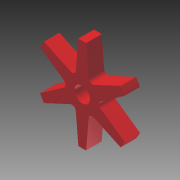
# Autodesk Inventor part: rubber intake star
Saved by Autodesk Inventor 2012 (Build 160160000, 160)
## iProperties
Created: 2013-07-07
Part Number: rubber intake star
Material: Default
Document SubType Name: Modeling
Designer: Bryce
Density: 1 g/cm^3
Author: Bryce
Autodesk Inventor part; units mm, degrees
ref_plane "YZ Plane" through (0, 0, 0) normal (1, 0, 0) x (0, 1, 0)
ref_plane "XZ Plane" through (0, 0, 0) normal (0, 1, 0) x (-1, 0, 0)
ref_plane "XY Plane" through (0, 0, 0) normal (0, 0, 1) x (1, 0, 0)
sketch "Sketch1" plane through (0, 0, 0) normal (0, 0, 1) x (1, 0, 0)
  arc A0 (3.175, 37.9675) -> (-3.175, 37.9675) centre (0, 0) ccw
  line L0 (-3.175, 37.9675) -> (-5.6418, 9.7719)
  line L1 (0, 38.1) -> (0, 0) construction
  arc A1 (-3.175, 37.9675) -> (-31.2933, 21.7334) centre (0, 0) ccw construction
  line L2 (-5.6418, 9.7719) -> (5.6418, 9.7719) construction
  line L3 (5.6418, 9.7719) -> (11.2836, 0) construction
  line L4 (11.2836, 0) -> (5.6418, -9.7719) construction
  line L5 (5.6418, -9.7719) -> (-5.6418, -9.7719) construction
  line L6 (-5.6418, -9.7719) -> (-11.2836, 0) construction
  line L7 (-11.2836, 0) -> (-5.6418, 9.7719) construction
  line L8 (3.175, 37.9675) -> (5.6418, 9.7719)
  line L9 (0, 0) -> (-32.9956, 19.05) construction
  line L10 (0, 0) -> (32.9956, 19.05) construction
  line L11 (0, 0) -> (-32.9956, -19.05) construction
  line L12 (0, 0) -> (32.9956, -19.05) construction
  line L13 (0, 0) -> (0, -38.1) construction
  line L14 (5.6418, 9.7719) -> (31.2933, 21.7334)
  line L15 (11.2836, 0) -> (34.4683, 16.2341)
  line L16 (11.2836, 0) -> (34.4683, -16.2341)
  line L17 (5.6418, -9.7719) -> (31.2933, -21.7334)
  arc A2 (31.2933, 21.7334) -> (3.175, 37.9675) centre (0, 0) ccw construction
  arc A3 (34.4683, 16.2341) -> (31.2933, 21.7334) centre (0, 0) ccw
  arc A4 (34.4683, -16.2341) -> (34.4683, 16.2341) centre (0, 0) ccw construction
  arc A5 (31.2933, -21.7334) -> (34.4683, -16.2341) centre (0, 0) ccw
  line L18 (5.6418, -9.7719) -> (3.175, -37.9675)
  line L19 (-5.6418, -9.7719) -> (-3.175, -37.9675)
  line L20 (-5.6418, -9.7719) -> (-31.2933, -21.7334)
  line L21 (-11.2836, 0) -> (-34.4683, -16.2341)
  line L22 (-11.2836, 0) -> (-34.4683, 16.2341)
  line L23 (-5.6418, 9.7719) -> (-31.2933, 21.7334)
  arc A6 (-31.2933, 21.7334) -> (-34.4683, 16.2341) centre (0, 0) ccw
  arc A7 (-34.4683, 16.2341) -> (-34.4683, -16.2341) centre (0, 0) ccw construction
  arc A8 (-34.4683, -16.2341) -> (-31.2933, -21.7334) centre (0, 0) ccw
  arc A9 (-31.2933, -21.7334) -> (-3.175, -37.9675) centre (0, 0) ccw construction
  arc A10 (-3.175, -37.9675) -> (3.175, -37.9675) centre (0, 0) ccw
  arc A11 (3.175, -37.9675) -> (31.2933, -21.7334) centre (0, 0) ccw construction
  circle A12 centre (0, 0) radius 6.35
  dimension "d10" = 38.1
  dimension "d1" = 6.35
  dimension "d2" = 3.175
  dimension "d3" = 5
  dimension "d5" = 5
  dimension "d6" = 5
  dimension "d7" = 5
  dimension "d8" = 5
  dimension "d9" = 5
  dimension "d13" = 12.7
  constraints: 48 end point, 47 point on circle, 10 centre point, 7 equal length, 3 coincident, 2 perpendicular, 1 collinear, 1 horizontal, 1 vertical, 49 other
  measures "d1" distance of L8.start L0.start
  measures "d2" horizontal distance of L1.start L0.start
  measures "d3" angle of L1 L0
  measures "d5" angle of L10 L14
  measures "d6" angle of L10 L15
  measures "d7" angle of L12 L16
  measures "d8" angle of L12 L17
  measures "d9" angle of L13 L19
  measures "d13" diameter of A12
extrude "Extrusion1" add sketch "Sketch1" along normal blind 12.7
fillet "Fillet1" radius 3.175 6 edges at (5.6418, 9.7719, 6.35) (-5.6418, 9.7719, 6.35) (-11.2836, 0, 6.35) (-5.6418, -9.7719, 6.35) (5.6418, -9.7719, 6.35) (11.2836, 0, 6.35)
equation "\"d2\" = 0.5 * d1"
equation "\"d5\" = d3"
equation "\"d6\" = d3"
equation "\"d8\" = d6"
equation "\"d9\" = d8"
body "Solid1"
